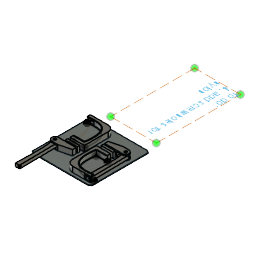
dipoledeployer_v2 (Autodesk Fusion 360 design; units mm, degrees)
Autodesk Fusion 360 part; units mm, degrees
sketch "Sketch1" plane through (0, 0, 0) normal (0, 0, 1) x (1, 0, 0) in component "baseplate"
  line L0 (0, 0) -> (100, 0)
  line L1 (100, 0) -> (100, -100)
  line L2 (100, -100) -> (0, -100)
  line L3 (0, -100) -> (0, 0)
  dimension "d1" = 100
  dimension "d2" = 100
  constraint horizontal L0
  constraint vertical L1
  constraint horizontal L2
  constraint vertical L3
  constraint coincident L0.start L3.end
  measures "d1" distance of L0.start L0.end
  measures "d2" distance of L0.start L2.end
extrude "Extrude1" add sketch "Sketch1" along normal blind 2 makes body 1 in component "baseplate"
sketch "Sketch2" plane through (0, 0, 2) normal (0, 0, 1) x (-1, 0, 0) in component "baseplate"
  line L0 (0, 100) -> (-100, 100)
  line L1 (-100, 100) -> (-100, 0)
  line L2 (-100, 0) -> (0, 0)
  line L3 (0, 0) -> (0, 100)
  line L4 (-50, 0) -> (-50, 100)
  line L5 (0, 50) -> (-100, 50)
  line L6 (-50, 50) -> (-50, 39)
  line L7 (-59, 29) -> (-79, 29)
  line L8 (-79, 29) -> (-79, 35)
  line L9 (-79, 35) -> (-59, 35)
  line L10 (-59, 35) -> (-59, 29)
  line L11 (-59, 37) -> (-79, 37)
  line L12 (-79, 37) -> (-79, 39)
  line L13 (-79, 39) -> (-59, 39)
  line L14 (-59, 39) -> (-59, 37)
  line L15 (-41, 29) -> (-21, 29)
  line L16 (-21, 29) -> (-21, 35)
  line L17 (-21, 35) -> (-41, 35)
  line L18 (-41, 35) -> (-41, 29)
  line L19 (-41, 37) -> (-21, 37)
  line L20 (-41, 39) -> (-41, 37)
  line L21 (-21, 39) -> (-41, 39)
  line L22 (-21, 37) -> (-21, 39)
  line L23 (-41, 71) -> (-21, 71)
  line L24 (-41, 65) -> (-41, 71)
  line L25 (-21, 65) -> (-41, 65)
  line L26 (-21, 71) -> (-21, 65)
  line L27 (-41, 63) -> (-21, 63)
  line L28 (-21, 61) -> (-41, 61)
  line L29 (-21, 63) -> (-21, 61)
  line L30 (-41, 61) -> (-41, 63)
  line L31 (-100, 0) -> (0, 100) construction
  line L32 (0, 0) -> (-100, 100) construction
  dimension "d5" = 20
  dimension "d6" = 6
  dimension "d7" = 9
  dimension "d8" = 15
  dimension "d11" = 2
  dimension "d12" = 20
  dimension "d13" = 2
  dimension "d14" = 9
  constraint midpoint L2 L4.start
  constraint midpoint L0 L4.end
  constraint midpoint L3 L5.start
  constraint midpoint L1 L5.end
  constraint midpoint L5 L6.start
  constraint coincident L4 L6.end
  constraint horizontal L7
  constraint vertical L8
  constraint horizontal L9
  constraint vertical L10
  constraint horizontal L11
  constraint vertical L12
  constraint horizontal L13
  constraint vertical L14
  constraint symmetric L4 L7.start L15.start
  constraint symmetric L4 L7.end L15.end
  constraint symmetric L4 L8.end L16.end
  constraint symmetric L4 L9.end L17.end
  constraint symmetric L4 L11.start L19.start
  constraint symmetric L4 L11.end L19.end
  constraint symmetric L4 L12.end L21.start
  constraint symmetric L4 L13.end L20.start
  constraint symmetric L5 L15.start L23.start
  constraint symmetric L5 L15.end L23.end
  constraint symmetric L5 L16.end L25.start
  constraint symmetric L5 L17.end L24.start
  constraint symmetric L5 L19.start L27.start
  constraint symmetric L5 L19.end L27.end
  constraint symmetric L5 L20.start L28.end
  constraint symmetric L5 L21.start L28.start
  constraint coincident L1.end L2.start
  constraint coincident L0.start L3.end
  constraint coincident L2.end L3.start
  constraint coincident L0.end L1.start
  measures "d5" distance of L7.start L7.end
  measures "d6" distance of L7.start L9.end
  measures "d7" distance of L4 L10
  measures "d8" distance of L5 L9
  measures "d11" distance of L9 L11
  measures "d12" distance of L12.end L13.end
  measures "d13" distance of L11.end L12.end
  measures "d14" distance of L4 L14
extrude "Extrude2" add sketch "Sketch2" along normal blind 15 separate body contours L7 L8 L9 L10 | L11 L12 L13 L14 makes body 2 at (65.6667, -29, 7) makes body 3 at (65.6667, -37, 7) in component "baseplate"
extrude "Extrude3" add sketch "Sketch2" along normal blind 15 contours L7 L8 L9 L10 | L11 L12 L13 L14 | L23 L24 L25 L26 | L27 L28 L29 L30 bodies 1 2 3 in component "baseplate"
sketch "Sketch3" plane through (0, -61, 0) normal (0, 1, 0) x (-1, 0, 0) in component "baseplate"
  line L0 (-41, 2) -> (-21, 2)
  line L1 (-21, 2) -> (-21, 17)
  line L2 (-21, 17) -> (-41, 17)
  line L3 (-41, 17) -> (-41, 2)
  line L4 (-21, 2) -> (-21, 9.5)
  line L5 (-21, 9.5) -> (-41, 9.5)
  line L6 (-31, 9.5) -> (-28, 9.5)
  circle A0 centre (-28, 9.5) radius 1.65
  line L7 (-31, 9.5) -> (-38, 9.5)
  circle A1 centre (-38, 9.5) radius 1.65
  dimension "d17" = 3.3
  dimension "d18" = 3.3
  constraint coincident L0.end L1.start
  constraint midpoint L1 L4.end
  constraint midpoint L3 L5.end
  constraint midpoint L5 L6.start
  constraint coincident L5 L6.end
  constraint coincident L6.end A0.centre
  constraint coincident L5 L7.end
  constraint coincident L7.end A1.centre
  measures "d17" diameter of A0
  measures "d18" diameter of A1
extrude "Extrude4" cut sketch "Sketch3" against normal blind 6 contours L5 L7 A1 | L5 L7 A1 | L5 L6 A0 | L5 L6 A0 bodies 1 in component "baseplate"
sketch "Sketch4" plane through (0, -39, 0) normal (0, -1, 0) x (1, 0, 0) in component "baseplate"
  line L0 (59, 2) -> (79, 2)
  line L1 (79, 2) -> (79, 17)
  line L2 (79, 17) -> (59, 17)
  line L3 (59, 17) -> (59, 2)
  line L4 (59, 17) -> (79, 2)
  line L5 (79, 17) -> (59, 2)
  line L6 (69, 9.5) -> (62, 9.5)
  line L7 (62, 9.5) -> (72, 9.5)
  circle A0 centre (62, 9.5) radius 1.65
  circle A1 centre (72, 9.5) radius 1.65
  dimension "d21" = 3.3
  dimension "d22" = 3.3
  constraint coincident L2.end L3.start
  constraint coincident L0.end L1.start
  constraint coincident L1.end L2.start
  constraint coincident L0.start L3.end
  constraint midpoint L4 L6.start
  constraint horizontal L6
  constraint parallel L6 L7
  constraint coincident L6.end L7.start
  constraint coincident L7.end A1.centre
  measures "d21" diameter of A0
  measures "d22" diameter of A1
extrude "Extrude5" cut sketch "Sketch4" against normal blind 6 contours A0 | A1 bodies 1 in component "baseplate"
sketch "Sketch5" plane through (0, 0, 2) normal (0, 0, 1) x (-1, 0, 0) in component "baseplate"
  line L0 (-21, 71) -> (-21, 65)
  line L1 (-21, 65) -> (-41, 65)
  line L2 (-41, 65) -> (-41, 71)
  line L3 (-41, 71) -> (-21, 71)
  line L4 (-59, 35) -> (-59, 29)
  line L5 (-59, 29) -> (-79, 29)
  line L6 (-79, 29) -> (-79, 35)
  line L7 (-79, 35) -> (-59, 35)
  line L8 (-41, 61) -> (-41, 63)
  line L9 (-41, 63) -> (-21, 63)
  line L10 (-21, 63) -> (-21, 61)
  line L11 (-21, 61) -> (-41, 61)
  line L12 (-59, 39) -> (-59, 37)
  line L13 (-59, 37) -> (-79, 37)
  line L14 (-79, 37) -> (-79, 39)
  line L15 (-79, 39) -> (-59, 39)
  line L16 (0, 100) -> (-100, 100)
  line L17 (-100, 100) -> (-100, 0)
  line L18 (-100, 0) -> (0, 0)
  line L19 (0, 0) -> (0, 100)
sketch "Sketch6" plane through (0, 0, 2) normal (0, 0, 1) x (-1, 0, 0) in component "baseplate"
  line L0 (-79, 35) -> (-89, 35)
  line L1 (-79, 29) -> (-79, 24)
  line L2 (-79, 24) -> (-89, 24)
  arc A0 (-89, 35) -> (-89, 24) centre (-89, 29.5) ccw
  line L3 (-21, 65) -> (-11, 65)
  line L4 (-21, 71) -> (-21, 76)
  line L5 (-21, 76) -> (-11, 76)
  arc A1 (-11, 65) -> (-11, 76) centre (-11, 70.5) ccw
  line L6 (-79, 24) -> (-59, 29)
  line L7 (-21, 76) -> (-41, 71)
  line L8 (-79, 35) -> (-79, 29)
  line L9 (-79, 29) -> (-59, 29)
  line L10 (-21, 71) -> (-21, 65)
  line L11 (-21, 71) -> (-41, 71)
  point P0 (-59, 29)
  point P1 (-41, 71)
  dimension "d33" = 10
  dimension "d34" = 5.5
  constraint horizontal L0
  constraint vertical L1
  constraint perpendicular L1 L2
  constraint tangent L0 A0
  constraint tangent L2 A0
  constraint horizontal L3
  constraint perpendicular L3 L4
  constraint perpendicular L4 L5
  constraint tangent L5 A1
  constraint tangent L3 A1
  constraint perpendicular L0 L8
  constraint perpendicular L1 L9
  constraint perpendicular L3 L10
  constraint perpendicular L4 L11
  constraint coincident P0 L6.end
  constraint coincident P1 L7.end
  measures "d33" distance of L0.start L0.end
  measures "d34" radius of A0
extrude "Extrude6" add sketch "Sketch6" along normal blind 15 bodies 1 in component "baseplate"
extrude "Extrude7" cut sketch "Sketch6" along normal blind 7 from surface at 4 contours L3 L4 L5 A1 L10 bodies 1 in component "baseplate"
extrude "Extrude8" cut sketch "Sketch6" along normal blind 7 from surface at 4 contours L0 L1 L2 A0 L8 bodies 1 in component "baseplate"
sketch "Sketch7" plane through (0, 0, 2) normal (0, 0, 1) x (-1, 0, 0) in component "baseplate"
  line L0 (-11, 65) -> (-41, 65)
  line L1 (-41, 65) -> (-41, 71)
  line L2 (-41, 71) -> (-21, 76)
  line L3 (-21, 76) -> (-11, 76)
  arc A0 (-11, 65) -> (-11, 76) centre (-11, 70.5) ccw
  line L4 (-89, 35) -> (-59, 35)
  line L5 (-59, 35) -> (-59, 29)
  line L6 (-59, 29) -> (-79, 24)
  line L7 (-79, 24) -> (-89, 24)
  arc A1 (-89, 35) -> (-89, 24) centre (-89, 29.5) ccw
  line L8 (-41, 61) -> (-41, 63)
  line L9 (-41, 63) -> (-21, 63)
  line L10 (-21, 63) -> (-21, 61)
  line L11 (-21, 61) -> (-41, 61)
  line L12 (-59, 39) -> (-59, 37)
  line L13 (-59, 37) -> (-79, 37)
  line L14 (-79, 37) -> (-79, 39)
  line L15 (-79, 39) -> (-59, 39)
  line L16 (0, 100) -> (-100, 100)
  line L17 (-100, 100) -> (-100, 0)
  line L18 (-100, 0) -> (0, 0)
  line L19 (0, 0) -> (0, 100)
sketch "Sketch8" plane through (0, 0, 17) normal (0, 0, 1) x (-1, 0, 0) in component "baseplate"
  line L0 (-41, 71) -> (-41, 65)
  line L1 (-41, 65) -> (-11, 65)
  arc A0 (-11, 65) -> (-11, 76) centre (-11, 70.5) ccw
  line L2 (-11, 76) -> (-21, 76)
  line L3 (-21, 76) -> (-41, 71)
  circle A1 centre (-11, 70.5) radius 2.25
  dimension "d35" = 4.5
  constraint concentric A0 A1
  measures "d35" diameter of A1
sketch "Sketch9" plane through (0, 0, 17) normal (0, 0, 1) x (-1, 0, 0) in component "baseplate"
  line L0 (-59, 35) -> (-89, 35)
  arc A0 (-89, 35) -> (-89, 24) centre (-89, 29.5) ccw
  line L1 (-89, 24) -> (-79, 24)
  line L2 (-79, 24) -> (-59, 29)
  line L3 (-59, 29) -> (-59, 35)
  circle A1 centre (-89, 29.5) radius 2.25
  dimension "d36" = 4.5
  constraint concentric A0 A1
  measures "d36" diameter of A1
extrude "Extrude9" cut sketch "Sketch9" sketch "Sketch8" against normal blind 15 contours A1 of sketch 2 contours A1 bodies 1 in component "baseplate"
sketch "Sketch10" plane through (0, 0, 2) normal (0, 0, 1) x (-1, 0, 0) in component "baseplate"
  line L0 (-79, 45) -> (-55, 45)
  line L1 (-55, 45) -> (-55, 85)
  line L2 (-65, 95) -> (-95, 95)
  line L3 (-95, 95) -> (-95, 90)
  line L4 (-79, 45) -> (-79, 50)
  arc A0 (-55, 85) -> (-65, 95) centre (-65, 85) ccw
  line L5 (-79, 50) -> (-60, 50)
  spline S0 degree 5 poles (-60, 50) (-59.7146, 51.8705) (-59.2285, 55.5196) (-58.7531, 60.7176) (-58.6353, 67.0874) (-59.4079, 74.0504) (-61.1872, 79.9198) (-64.0631, 84.5979) (-68.0975, 88.0173) (-73.2633, 90.2075) (-79.4828, 91.2531) (-85.236, 91.2448) (-89.961, 90.7929) (-93.2905, 90.2968) (-95, 90) knots 0 0 0 0 0 0 0.1 0.2 0.3 0.4 0.5 0.6 0.7 0.8 0.9 1 1 1 1 1 1
  line L6 (-50, 0) -> (-50, 100)
  line L7 (-21, 45) -> (-45, 45)
  line L8 (-21, 45) -> (-21, 50)
  line L9 (-21, 50) -> (-40, 50)
  spline S1 degree 5 poles (-40, 50) (-40.2854, 51.8705) (-40.7715, 55.5196) (-41.2469, 60.7176) (-41.3647, 67.0874) (-40.5921, 74.0504) (-38.8128, 79.9198) (-35.9369, 84.5979) (-31.9025, 88.0173) (-26.7367, 90.2075) (-20.5172, 91.2531) (-14.764, 91.2448) (-10.039, 90.7929) (-6.7095, 90.2968) (-5, 90) knots 0 0 0 0 0 0 0.1 0.2 0.3 0.4 0.5 0.6 0.7 0.8 0.9 1 1 1 1 1 1
  line L10 (-61.5241, 40.0105) -> (-58.4759, 59.9895)
  line L11 (-85.1973, 91.7017) -> (-104.8027, 88.2983)
  line L12 (-38.4759, 40.0105) -> (-41.5241, 59.9895)
  line L13 (-14.8027, 91.7017) -> (4.8027, 88.2983)
  line L14 (-45, 45) -> (-45, 85)
  arc A1 (-35, 95) -> (-45, 85) centre (-35, 85) ccw
  line L15 (-35, 95) -> (-5, 95)
  line L16 (-5, 95) -> (-5, 90)
  line L17 (0, 50) -> (-100, 50)
  line L18 (-21, 55) -> (-45, 55)
  line L19 (-45, 55) -> (-45, 15)
  line L20 (-21, 55) -> (-21, 50)
  line L21 (-21, 50) -> (-40, 50)
  spline S2 degree 5 poles (-40, 50) (-40.2854, 48.1295) (-40.7715, 44.4804) (-41.2469, 39.2824) (-41.3647, 32.9126) (-40.5921, 25.9496) (-38.8128, 20.0802) (-35.9369, 15.4021) (-31.9025, 11.9827) (-26.7367, 9.7925) (-20.5172, 8.7469) (-14.764, 8.7552) (-10.039, 9.2071) (-6.7095, 9.7032) (-5, 10) knots 0 0 0 0 0 0 0.1 0.2 0.3 0.4 0.5 0.6 0.7 0.8 0.9 1 1 1 1 1 1
  line L22 (-38.4759, 59.9895) -> (-41.5241, 40.0105)
  line L23 (-14.8027, 8.2983) -> (4.8027, 11.7017)
  arc A2 (-45, 15) -> (-35, 5) centre (-35, 15) ccw
  line L24 (-35, 5) -> (-5, 5)
  line L25 (-5, 5) -> (-5, 10)
  point P0 (-65, 85)
  point P1 (-35, 85)
  point P2 (-35, 15)
  dimension "d39" = 24
  dimension "d40" = 5
  dimension "d41" = 5
  dimension "d42" = 10
  dimension "d43" = 40
  dimension "d44" = 30
  dimension "d45" = 19
  constraint horizontal L0
  constraint perpendicular L0 L1
  constraint perpendicular L1 L2
  constraint perpendicular L2 L3
  constraint perpendicular L0 L4
  constraint tangent L1 A0
  constraint tangent L2 A0
  constraint perpendicular L4 L5
  constraint coincident P0 A0.centre
  constraint midpoint L5.end L10
  constraint midpoint L3.end L11
  constraint symmetric L0.start L6 L7.start
  constraint symmetric L0.end L6 L7.end
  constraint symmetric L2.end L6 L15.end
  constraint symmetric L3.end L6 S1.end
  constraint symmetric L4.end L6 L8.end
  constraint symmetric L1.end L6 L14.end
  constraint symmetric L2.start L6 A1.start
  constraint symmetric A0 L6 A1
  constraint symmetric L5.end L6 L9.end
  constraint symmetric P0 L6 P1
  constraint symmetric L6 L10.start L12.start
  constraint symmetric L6 L10.end L12.end
  constraint symmetric L6 L11.start L13.start
  constraint symmetric L6 L11.end L13.end
  constraint symmetric L7.start L17 L18.start
  constraint symmetric L7.end L17 L18.end
  constraint symmetric L8.end L17 L9.start
  constraint symmetric L9.end L17 S1.start
  constraint symmetric P1 L17 P2
  constraint symmetric S1.end L17 S2.end
  constraint symmetric L12.start L17 L22.start
  constraint symmetric L12.end L17 L22.end
  constraint symmetric L13.start L17 L23.start
  constraint symmetric L13.end L17 L23.end
  constraint symmetric L14.end L17 L19.end
  constraint symmetric A1.start L17 A2.end
  constraint symmetric A1 L17 A2
  constraint symmetric L15.end L17 L24.end
  measures "d39" distance of L0.start L0.end
  measures "d40" distance of L2.end L3.end
  measures "d41" distance of L0.start L4.end
  measures "d42" radius of A0
  measures "d43" distance of L0.end L1.end
  measures "d44" distance of L2.end L2.start
  measures "d45" distance of L4.end L5.end
extrude "Extrude10" add sketch "Sketch10" along normal blind 15 contours L0 L4 L5 L10 L17 | L0 L1 L10 L17 | L1 L2 L3 A0 S0 L17 | L9 L17 L18 L20 L21 L22 | L7 L19 S2 A2 L24 L25 | L7 S2 L22 | S1 L12 L18 | L12 L14 L17 L18 L19 | L7 L14 L17 L19 L22 | S1 L18 L22 bodies 1 in component "baseplate"
sketch "Sketch11" plane through (0, 0, 17) normal (0, 0, 1) x (-1, 0, 0) in component "baseplate"
  line L0 (-79, 45) -> (-55, 45)
  line L1 (-55, 45) -> (-55, 85)
  arc A0 (-55, 85) -> (-65, 95) centre (-65, 85) ccw
  line L2 (-65, 95) -> (-95, 95)
  line L3 (-95, 95) -> (-95, 90)
  spline S0 degree 5 poles (-95, 90) (-93.2905, 90.2968) (-89.961, 90.7929) (-85.236, 91.2448) (-79.4828, 91.2531) (-73.2633, 90.2075) (-68.0975, 88.0173) (-64.0631, 84.5979) (-61.1872, 79.9198) (-59.4079, 74.0504) (-58.6353, 67.0874) (-58.7531, 60.7176) (-59.2285, 55.5196) (-59.7146, 51.8705) (-60, 50) knots -1 -1 -1 -1 -1 -1 -0.9 -0.8 -0.7 -0.6 -0.5 -0.4 -0.3 -0.2 -0.1 0 0 0 0 0 0
  line L4 (-60, 50) -> (-79, 50)
  line L5 (-79, 50) -> (-79, 45)
  line L6 (-95, 95) -> (-85, 95)
  line L7 (-85, 95) -> (-85, 91.0896)
  line L8 (-5, 5) -> (-15, 5)
  line L9 (-15, 5) -> (-15, 9)
  line L10 (-5, 5) -> (-5, 10)
  line L11 (-5, 10) -> (-15, 10)
  line L12 (-15, 10) -> (-15, 9)
  dimension "d48" = 10
  dimension "d49" = 90
  dimension "d50" = 10
  constraint coincident L2.end L3.start
  constraint perpendicular L3 L6
  constraint coincident S0 L7.end
  constraint perpendicular L6 L7
  constraint perpendicular L8 L9
  constraint perpendicular L8 L10
  constraint perpendicular L10 L11
  measures "d48" distance of L2.end L6.end
  measures "d49" angle of L7 L8
  measures "d50" distance of L8.start L8.end
extrude "Extrude11" cut sketch "Sketch11" against normal blind 7 from surface at -4 contours L2 L3 S0 L6 L7 | L8 L9 L10 L11 L12 bodies 1 in component "baseplate"
sketch "Sketch13" plane through (0, 0, 6) normal (0, 0, 1) x (-1, 0, 0) in component "baseplate"
  circle A0 centre (-11, 70.5) radius 2.25
  line L0 (-21, 76) -> (-21, 65)
  line L1 (-21, 65) -> (-11, 65)
  arc A1 (-11, 65) -> (-11, 76) centre (-11, 70.5) ccw
  line L2 (-11, 76) -> (-21, 76)
  circle A2 centre (-11, 70.5) radius 5
  line L3 (-5, 5) -> (-6.0006, 70.5763)
  line L4 (-5, 5) -> (-11.9992, 4.8932)
  spline S0 degree 5 poles (-11.9992, 4.8932) (-11.9252, 6.9328) (-11.7854, 10.9544) (-11.6002, 16.8138) (-11.4027, 24.2745) (-11.2457, 32.964) (-11.1908, 40.9291) (-11.255, 48.049) (-11.4586, 54.1813) (-11.821, 59.1863) (-12.3579, 62.9548) (-12.9282, 64.9707) (-13.4323, 65.9409) (-13.8018, 66.3506) (-13.9949, 66.4962) knots 0 0 0 0 0 0 0.1 0.2 0.3 0.4 0.5 0.6 0.7 0.8 0.9 1 1 1 1 1 1
  point P0 (-11.9992, 60.0714)
  dimension "d54" = 10
  dimension "d55" = 7
  constraint concentric A0 A2
  constraint coincident A2 L3.end
  constraint tangent A2 L3
  constraint perpendicular L3 L4
  constraint coincident A2 S0.end
  measures "d54" diameter of A2
  measures "d55" distance of L3.start L4.end
extrude "Extrude1'" add sketch "Sketch13" along normal blind 6.5 from surface at 0.25 separate body contours L1 A1 A2 L3 S0 | L1 A1 L3 L4 S0 | A2 L3 sketch seen with x (1, 0, 0) y (0, 1, 0) z (0, 0, 1) at (0.3158, -2.7195, 1.082) makes body 4
copy_body "CopyPasteBodies1" bodies 4 makes body 5
move_body "Move1" bodies 5 to x (-1, 0, 0) y (0, -1, 0) z (0, 0, 1) at (100.6316, -105.4389, 0)
copy_body "Body->Comp1" bodies 4 removing the originals makes body 6 in component "arm1"
copy_body "Body->Comp2" bodies 5 removing the originals makes body 7 in component "arm2"
sketch "Sketch1 (2)" plane through (0, 0, 3.082) normal (0, 0, 1) x (-1, 0, 0)
  line L0 (-21.3158, 57.7195) -> (-21.3158, 52.7195)
  line L1 (-21.3158, 52.7195) -> (-40.3158, 52.7195)
  spline S0 degree 5 poles (-40.3158, 52.7195) (-40.6012, 50.8489) (-41.0873, 47.1998) (-41.5627, 42.0019) (-41.6805, 35.632) (-40.9079, 28.669) (-39.1286, 22.7997) (-36.2527, 18.1216) (-32.2183, 14.7022) (-27.0525, 12.5119) (-20.833, 11.4663) (-15.0798, 11.4747) (-10.3547, 11.9266) (-7.0253, 12.4227) (-5.3158, 12.7195) knots 0 0 0 0 0 0 0.1 0.2 0.3 0.4 0.5 0.6 0.7 0.8 0.9 1 1 1 1 1 1
  line L2 (-5.3158, 12.7195) -> (-5.3158, 7.7195)
  line L3 (-5.3158, 7.7195) -> (-35.3158, 7.7195)
  arc A0 (-45.3158, 17.7195) -> (-35.3158, 7.7195) centre (-35.3158, 17.7195) ccw
  line L4 (-45.3158, 17.7195) -> (-45.3158, 57.7195)
  line L5 (-45.3158, 57.7195) -> (-21.3158, 57.7195)
  line L6 (-79.3158, 47.7195) -> (-79.3158, 52.7195)
  line L7 (-79.3158, 52.7195) -> (-60.3158, 52.7195)
  spline S1 degree 5 poles (-60.3158, 52.7195) (-60.0304, 54.59) (-59.5443, 58.2391) (-59.0688, 63.437) (-58.9511, 69.8069) (-59.7237, 76.7699) (-61.503, 82.6392) (-64.3788, 87.3173) (-68.4133, 90.7368) (-73.5791, 92.927) (-79.7986, 93.9726) (-85.5518, 93.9642) (-90.2768, 93.5123) (-93.6062, 93.0162) (-95.3158, 92.7195) knots 0 0 0 0 0 0 0.1 0.2 0.3 0.4 0.5 0.6 0.7 0.8 0.9 1 1 1 1 1 1
  line L8 (-95.3158, 92.7195) -> (-95.3158, 97.7195)
  line L9 (-95.3158, 97.7195) -> (-65.3158, 97.7195)
  arc A1 (-55.3158, 87.7195) -> (-65.3158, 97.7195) centre (-65.3158, 87.7195) ccw
  line L10 (-55.3158, 87.7195) -> (-55.3158, 47.7195)
  line L11 (-55.3158, 47.7195) -> (-79.3158, 47.7195)
  line L12 (-11.3158, 67.7195) -> (-41.3158, 67.7195)
  line L13 (-41.3158, 67.7195) -> (-41.3158, 73.7195)
  line L14 (-41.3158, 73.7195) -> (-21.3158, 78.7195)
  line L15 (-21.3158, 78.7195) -> (-11.3158, 78.7195)
  arc A2 (-11.3158, 67.7195) -> (-11.3158, 78.7195) centre (-11.3158, 73.2195) ccw
  line L16 (-89.3158, 37.7195) -> (-59.3158, 37.7195)
  line L17 (-59.3158, 37.7195) -> (-59.3158, 31.7195)
  line L18 (-59.3158, 31.7195) -> (-79.3158, 26.7195)
  line L19 (-79.3158, 26.7195) -> (-89.3158, 26.7195)
  arc A3 (-89.3158, 37.7195) -> (-89.3158, 26.7195) centre (-89.3158, 32.2195) ccw
  line L20 (-41.3158, 63.7195) -> (-41.3158, 65.7195)
  line L21 (-41.3158, 65.7195) -> (-21.3158, 65.7195)
  line L22 (-21.3158, 65.7195) -> (-21.3158, 63.7195)
  line L23 (-21.3158, 63.7195) -> (-41.3158, 63.7195)
  line L24 (-59.3158, 41.7195) -> (-59.3158, 39.7195)
  line L25 (-59.3158, 39.7195) -> (-79.3158, 39.7195)
  line L26 (-79.3158, 39.7195) -> (-79.3158, 41.7195)
  line L27 (-79.3158, 41.7195) -> (-59.3158, 41.7195)
  line L28 (-0.3158, 102.7195) -> (-100.3158, 102.7195)
  line L29 (-100.3158, 102.7195) -> (-100.3158, 2.7195)
  line L30 (-100.3158, 2.7195) -> (-0.3158, 2.7195)
  line L31 (-0.3158, 2.7195) -> (-0.3158, 102.7195)
sketch "Sketch14" plane through (0, 0, 2) normal (0, 0, 1) x (-1, 0, 0) in component "baseplate"
  line L0 (-50, 50) -> (-47.8211, 74.9049)
  line L1 (-50, 50) -> (-25, 50) construction
  circle A0 centre (-47.8211, 74.9049) radius 2.5
  line L2 (-47.8211, 74.9049) -> (-52.1789, 25.0951)
  circle A1 centre (-52.1789, 25.0951) radius 2.5
  dimension "d68" = 85
  dimension "d69" = 25
  dimension "d70" = 5
  dimension "d71" = 50
  dimension "d72" = 5
  constraint horizontal L1
  constraint coincident L0.end A0.centre
  constraint parallel L0 L2
  constraint coincident L2.end A1.centre
  measures "d68" angle of L0 L1
  measures "d69" distance of L0.start L0.end
  measures "d70" diameter of A0
  measures "d71" distance of L0.end L2.end
  measures "d72" diameter of A1
extrude "Extrude15" cut sketch "Sketch14" against normal blind 2 bodies 1 in component "baseplate"
sketch "Sketch2 (2)" plane through (0, 0, 13.832) normal (0, 0, 1) x (-1, 0, 0)
  circle A0 centre (-89.3158, 32.2195) radius 2.25
  line L0 (-95.3158, 97.7195) -> (-94.3152, 32.1432)
  arc A1 (-94.3152, 32.1432) -> (-86.3209, 36.2233) centre (-89.3158, 32.2195) ccw
  spline S0 degree 5 poles (-86.3209, 36.2233) (-86.514, 36.3689) (-86.8835, 36.7786) (-87.3876, 37.7488) (-87.9579, 39.7647) (-88.4948, 43.5331) (-88.8572, 48.5382) (-89.0608, 54.6705) (-89.125, 61.7904) (-89.0701, 69.7554) (-88.9131, 78.4449) (-88.7156, 85.9057) (-88.5303, 91.7651) (-88.3906, 95.7866) (-88.3166, 97.8263) knots -1 -1 -1 -1 -1 -1 -0.9 -0.8 -0.7 -0.6 -0.5 -0.4 -0.3 -0.2 -0.1 0 0 0 0 0 0
  line L1 (-88.3166, 97.8263) -> (-95.3158, 97.7195)
sketch "Sketch2 (3)" plane through (0, 0, 13.832) normal (0, 0, 1) x (-1, 0, 0) in component "arm2"
  circle A0 centre (-89.3158, 32.2195) radius 2.25
  line L0 (-95.3158, 97.7195) -> (-94.3152, 32.1432)
  arc A1 (-94.3152, 32.1432) -> (-86.3209, 36.2233) centre (-89.3158, 32.2195) ccw
  spline S0 degree 5 poles (-86.3209, 36.2233) (-86.514, 36.3689) (-86.8835, 36.7786) (-87.3876, 37.7488) (-87.9579, 39.7647) (-88.4948, 43.5331) (-88.8572, 48.5382) (-89.0608, 54.6705) (-89.125, 61.7904) (-89.0701, 69.7554) (-88.9131, 78.4449) (-88.7156, 85.9057) (-88.5303, 91.7651) (-88.3906, 95.7866) (-88.3166, 97.8263) knots -1 -1 -1 -1 -1 -1 -0.9 -0.8 -0.7 -0.6 -0.5 -0.4 -0.3 -0.2 -0.1 0 0 0 0 0 0
  line L1 (-88.3166, 97.8263) -> (-95.3158, 97.7195)
  line L2 (-95.3158, 97.7195) -> (-95.27, 94.7198)
  line L3 (-95.3158, 97.7195) -> (-92.3161, 97.7652)
  line L4 (-92.3161, 97.7652) -> (-95.27, 94.7198)
  dimension "d89" = 3
  dimension "d90" = 3
  constraint coincident L0.start L1.end
  constraint perpendicular L1 L2
  constraint coincident L1 L3.end
  measures "d89" distance of L0.start L2.end
  measures "d90" distance of L0.start L3.end
extrude "Extrude1''" cut sketch "Sketch2 (3)" against normal blind 1 from surface at -3 contours L0 L1 L2 L3 L4 bodies 7 in component "arm2"
sketch "Sketch1 (3)" plane through (0, 0, 13.832) normal (0, 0, 1) x (-1, 0, 0) in component "arm1"
  circle A0 centre (-11.3158, 73.2195) radius 2.25
  line L0 (-5.3158, 7.7195) -> (-6.3164, 73.2957)
  arc A1 (-6.3164, 73.2957) -> (-14.3107, 69.2157) centre (-11.3158, 73.2195) ccw
  spline S0 degree 5 poles (-14.3107, 69.2157) (-14.1176, 69.0701) (-13.7481, 68.6604) (-13.244, 67.6902) (-12.6737, 65.6742) (-12.1368, 61.9058) (-11.7743, 56.9007) (-11.5708, 50.7684) (-11.5066, 43.6485) (-11.5615, 35.6835) (-11.7185, 26.994) (-11.916, 19.5332) (-12.1012, 13.6739) (-12.241, 9.6523) (-12.315, 7.6127) knots -1 -1 -1 -1 -1 -1 -0.9 -0.8 -0.7 -0.6 -0.5 -0.4 -0.3 -0.2 -0.1 0 0 0 0 0 0
  line L1 (-12.315, 7.6127) -> (-5.3158, 7.7195)
  line L2 (-5.3158, 7.7195) -> (-5.3616, 10.7191)
  line L3 (-5.3158, 7.7195) -> (-8.3154, 7.6737)
  line L4 (-8.3154, 7.6737) -> (-5.3616, 10.7191)
  dimension "d94" = 3
  dimension "d95" = 3
  constraint coincident L0.start L1.end
  constraint perpendicular L1 L2
  constraint perpendicular L2 L3
  measures "d94" distance of L0.start L2.end
  measures "d95" distance of L0.start L3.end
extrude "Extrude1'''" cut sketch "Sketch1 (3)" against normal blind 1 from surface at -3 contours L0 L1 L2 L3 L4 bodies 6 in component "arm1"
sketch "Sketch15" plane through (-0.3158, 2.7195, 2) normal (0, 0, 1) x (-1, 0, 0) in component "baseplate"
  circle A0 centre (-52.4947, 27.8146) radius 2.5
  circle A1 centre (-48.1369, 77.6243) radius 2.5
  line L0 (-21.3158, 57.7195) -> (-21.3158, 52.7195)
  line L1 (-21.3158, 52.7195) -> (-40.3158, 52.7195)
  spline S0 degree 5 poles (-40.3158, 52.7195) (-40.6012, 50.8489) (-41.0873, 47.1998) (-41.5627, 42.0019) (-41.6805, 35.632) (-40.9079, 28.669) (-39.1286, 22.7997) (-36.2527, 18.1216) (-32.2183, 14.7022) (-27.0525, 12.5119) (-20.833, 11.4663) (-15.0798, 11.4747) (-10.3547, 11.9266) (-7.0253, 12.4227) (-5.3158, 12.7195) knots 0 0 0 0 0 0 0.1 0.2 0.3 0.4 0.5 0.6 0.7 0.8 0.9 1 1 1 1 1 1
  line L2 (-5.3158, 12.7195) -> (-5.3158, 7.7195)
  line L3 (-5.3158, 7.7195) -> (-35.3158, 7.7195)
  arc A2 (-45.3158, 17.7195) -> (-35.3158, 7.7195) centre (-35.3158, 17.7195) ccw
  line L4 (-45.3158, 17.7195) -> (-45.3158, 57.7195)
  line L5 (-45.3158, 57.7195) -> (-21.3158, 57.7195)
  line L6 (-79.3158, 47.7195) -> (-79.3158, 52.7195)
  line L7 (-79.3158, 52.7195) -> (-60.3158, 52.7195)
  spline S1 degree 5 poles (-60.3158, 52.7195) (-60.0304, 54.59) (-59.5443, 58.2391) (-59.0688, 63.437) (-58.9511, 69.8069) (-59.7237, 76.7699) (-61.503, 82.6392) (-64.3788, 87.3173) (-68.4133, 90.7368) (-73.5791, 92.927) (-79.7986, 93.9726) (-85.5518, 93.9642) (-90.2768, 93.5123) (-93.6062, 93.0162) (-95.3158, 92.7195) knots 0 0 0 0 0 0 0.1 0.2 0.3 0.4 0.5 0.6 0.7 0.8 0.9 1 1 1 1 1 1
  line L8 (-95.3158, 92.7195) -> (-95.3158, 97.7195)
  line L9 (-95.3158, 97.7195) -> (-65.3158, 97.7195)
  arc A3 (-55.3158, 87.7195) -> (-65.3158, 97.7195) centre (-65.3158, 87.7195) ccw
  line L10 (-55.3158, 87.7195) -> (-55.3158, 47.7195)
  line L11 (-55.3158, 47.7195) -> (-79.3158, 47.7195)
  line L12 (-11.3158, 67.7195) -> (-41.3158, 67.7195)
  line L13 (-41.3158, 67.7195) -> (-41.3158, 73.7195)
  line L14 (-41.3158, 73.7195) -> (-21.3158, 78.7195)
  line L15 (-21.3158, 78.7195) -> (-11.3158, 78.7195)
  arc A4 (-11.3158, 67.7195) -> (-11.3158, 78.7195) centre (-11.3158, 73.2195) ccw
  line L16 (-89.3158, 37.7195) -> (-59.3158, 37.7195)
  line L17 (-59.3158, 37.7195) -> (-59.3158, 31.7195)
  line L18 (-59.3158, 31.7195) -> (-79.3158, 26.7195)
  line L19 (-79.3158, 26.7195) -> (-89.3158, 26.7195)
  arc A5 (-89.3158, 37.7195) -> (-89.3158, 26.7195) centre (-89.3158, 32.2195) ccw
  line L20 (-41.3158, 63.7195) -> (-41.3158, 65.7195)
  line L21 (-41.3158, 65.7195) -> (-21.3158, 65.7195)
  line L22 (-21.3158, 65.7195) -> (-21.3158, 63.7195)
  line L23 (-21.3158, 63.7195) -> (-41.3158, 63.7195)
  line L24 (-59.3158, 41.7195) -> (-59.3158, 39.7195)
  line L25 (-59.3158, 39.7195) -> (-79.3158, 39.7195)
  line L26 (-79.3158, 39.7195) -> (-79.3158, 41.7195)
  line L27 (-79.3158, 41.7195) -> (-59.3158, 41.7195)
  line L28 (-0.3158, 102.7195) -> (-100.3158, 102.7195)
  line L29 (-100.3158, 102.7195) -> (-100.3158, 2.7195)
  line L30 (-100.3158, 2.7195) -> (-0.3158, 2.7195)
  line L31 (-0.3158, 2.7195) -> (-0.3158, 102.7195)
  line L32 (-0.3158, 2.7195) -> (-2.3158, 2.7195)
  line L33 (-2.3158, 2.7195) -> (-2.3158, 4.7195)
  line L34 (-2.3158, 4.7195) -> (-0.3158, 4.7195)
  line L35 (-0.3158, 4.7195) -> (-0.3158, 2.7195)
  line L36 (-2.3158, 4.7195) -> (-4.3158, 2.7195)
  line L37 (-2.3158, 4.7195) -> (0.5126, 4.7195) construction
  line L38 (-2.3158, 2.7195) -> (-4.3158, 2.7195)
  line L39 (-50.3158, 2.7195) -> (-50.3158, 102.7195)
  line L40 (-98.3158, 4.7195) -> (-96.3158, 2.7195)
  line L41 (-98.3158, 2.7195) -> (-98.3158, 4.7195)
  line L42 (-98.3158, 2.7195) -> (-96.3158, 2.7195)
  line L43 (-100.3158, 2.7195) -> (-98.3158, 2.7195)
  line L44 (-100.3158, 4.7195) -> (-100.3158, 2.7195)
  line L45 (-98.3158, 4.7195) -> (-100.3158, 4.7195)
  line L46 (-0.3158, 52.7195) -> (-100.3158, 52.7195)
  line L47 (-100.3158, 102.7195) -> (-98.3158, 102.7195)
  line L48 (-98.3158, 102.7195) -> (-96.3158, 102.7195)
  line L49 (-98.3158, 100.7195) -> (-96.3158, 102.7195)
  line L50 (-98.3158, 102.7195) -> (-98.3158, 100.7195)
  line L51 (-98.3158, 100.7195) -> (-100.3158, 100.7195)
  line L52 (-100.3158, 100.7195) -> (-100.3158, 102.7195)
  line L53 (-2.3158, 100.7195) -> (-4.3158, 102.7195)
  line L54 (-2.3158, 102.7195) -> (-4.3158, 102.7195)
  line L55 (-2.3158, 102.7195) -> (-2.3158, 100.7195)
  line L56 (-0.3158, 102.7195) -> (-2.3158, 102.7195)
  line L57 (-0.3158, 100.7195) -> (-0.3158, 102.7195)
  line L58 (-2.3158, 100.7195) -> (-0.3158, 100.7195)
  dimension "d99" = 2
  dimension "d100" = 2
  dimension "d101" = 135
  constraint horizontal L32
  constraint vertical L33
  constraint horizontal L34
  constraint vertical L35
  constraint coincident L30.end L31.start
  constraint horizontal L37
  constraint coincident L30 L36.end
  constraint symmetric L30.end L39 L29.end
  constraint symmetric L32.end L39 L41.start
  constraint symmetric L33.end L39 L40.start
  constraint symmetric L34.end L39 L44.start
  constraint symmetric L36.end L39 L40.end
  constraint symmetric L30.end L46 L28.start
  constraint symmetric L32.end L46 L54.start
  constraint symmetric L33.end L46 L53.start
  constraint symmetric L34.end L46 L57.start
  constraint symmetric L36.end L46 L53.end
  constraint symmetric L40.start L46 L49.start
  constraint symmetric L40.end L46 L48.end
  constraint symmetric L41.start L46 L47.end
  constraint symmetric L29.end L46 L28.end
  constraint symmetric L44.start L46 L51.end
  measures "d99" distance of L30.end L32.end
  measures "d100" distance of L30.end L34.end
  measures "d101" angle of L36 L37
extrude "Extrude16" cut sketch "Sketch15" against normal blind 6 contours L30 L40 L41 L42 | L30 L33 L36 L38 | L29 L30 L41 L43 L44 L45 | L30 L31 L32 L33 L34 L35 | L28 L53 L54 L55 | L28 L48 L49 L50 | L28 L31 L55 L56 L57 L58 | L28 L29 L47 L50 L51 L52 bodies 1 in component "baseplate"
extrude "Extrude17" cut 1 faces at (16.5229, -57.9401, 0) along direction (0, 0, 1) blind 0.5 on bodies 1 bodies 1 in component "baseplate"
extrude "Extrude19" add 1 faces at (30.1224, -61, 3.9638) along direction (0, 1, 0) blind 2 on bodies 1 bodies 1 in component "baseplate"
sketch "Sketch4 (2)" plane through (0, 0, 0) normal (0, 0, 1) x (1, 0, 0)
  line L0 (13.0179, 160) -> (13.0179, 18.7039) construction
  line L1 (13.0179, 18.7039) -> (90, 18.7039) construction
  line L2 (90, 18.7039) -> (90, 160) construction
  line L3 (90, 160) -> (13.0179, 160) construction
  dimension "d110" = 10
extrude "Extrude20" cut 4 faces at (18.4167, -70.5, 6) (10.0636, -6.4202, 6) (81.5833, -29.5, 6) (89.9407, -93.5793, 6) along direction (0, 0, -1) blind 2.75 on bodies 1 bodies 1 in component "baseplate"
extrude "Extrude21" add 4 faces at (81.5833, -29.5, 13) (89.9407, -93.5793, 13) (10.0636, -6.4202, 13) (18.4167, -70.5, 13) along direction (0, 0, -1) blind 3.75 on bodies 1 bodies 1 in component "baseplate"
extrude "Extrude22" cut 6 faces at (35.3333, -53.3333, 17) (24.953, -70.0775, 17) (27.6667, -60.3333, 17) (65.6667, -37.6667, 17) (64.6667, -46.6667, 17) (75.047, -29.9225, 17) along direction (0, 0, -1) blind 5.75 on bodies 1 bodies 1 in component "baseplate"
extrude "Extrude2'" cut 1 faces at (9.7227, -19.8097, 13.832) along direction (0, 0, -1) blind 1 on bodies 6 bodies 6 in component "arm1"
extrude "Extrude3'" cut 1 faces at (6.3309, -8.7041, 9.832) along direction (0, 0, -1) blind 0.5 on bodies 6 bodies 6 in component "arm1"
extrude "Extrude23" cut 1 faces at (16.5229, -57.9401, 0.5) along direction (0, 0, 1) blind 0.5 on bodies 1 bodies 1 in component "baseplate"
extrude "Extrude24" cut 1 faces at (16.5229, -57.9401, 1) along direction (0, 0, 1) blind 0.25 on bodies 1 bodies 1 in component "baseplate"
delete_face "DeleteFace2" 1 faces at (72.6786, -38.3333, 7.996) on bodies 1 in component "baseplate"
delete_face "DeleteFace3" 1 faces at (61.1048, -37.6667, 8.114) on bodies 1 in component "baseplate"
delete_face "DeleteFace4" 1 faces at (61.1048, -33.6667, 8.114) on bodies 1 in component "baseplate"
delete_face "DeleteFace5" 1 faces at (71.2473, -33.6667, 8.0317) on bodies 1 in component "baseplate"
delete_face "DeleteFace6" 1 faces at (38.8952, -61.6667, 8.114) on bodies 1 in component "baseplate"
delete_face "DeleteFace7" 1 faces at (26.3521, -60.3333, 9.5822) on bodies 1 in component "baseplate"
delete_face "DeleteFace8" 1 faces at (26.3521, -66.3333, 9.4178) on bodies 1 in component "baseplate"
delete_face "DeleteFace9" 1 faces at (38.8952, -66.3333, 8.114) on bodies 1 in component "baseplate"
extrude "Extrude25" add 1 faces at (72.3333, -39, 5.0833) along direction (0, -1, 0) blind 2 on bodies 1 bodies 1 in component "baseplate"
sketch "Sketch6 (2)" plane through (0, 0, -1.7946) normal (0, 0, 1) x (-1, 0, 0)
  circle A0 centre (-173.3503, 9.3964) radius 2.25
  line L0 (-179.3503, 74.8964) -> (-178.3497, 9.3201)
  arc A1 (-178.3497, 9.3201) -> (-170.3553, 13.4002) centre (-173.3503, 9.3964) ccw
  spline S0 degree 5 poles (-170.3553, 13.4002) (-170.5484, 13.5458) (-170.918, 13.9555) (-171.4221, 14.9257) (-171.9924, 16.9416) (-172.5292, 20.7101) (-172.8917, 25.7151) (-173.0952, 31.8474) (-173.1595, 38.9673) (-173.1046, 46.9324) (-172.9475, 55.6219) (-172.7501, 63.0826) (-172.5648, 68.942) (-172.425, 72.9635) (-172.3511, 75.0032) knots -1 -1 -1 -1 -1 -1 -0.9 -0.8 -0.7 -0.6 -0.5 -0.4 -0.3 -0.2 -0.1 0 0 0 0 0 0
  line L1 (-172.3511, 75.0032) -> (-179.3503, 74.8964)
  line L2 (-178.3695, 10.6201) -> (-175.1888, 4.7466)
  line L3 (-178.3695, 10.6201) -> (-183.3265, 4.9429)
  line L4 (-183.3265, 4.9429) -> (-175.1888, 4.7466)
  constraint coincident L0 L2.start
  constraint coincident A1 L2.end
extrude "Extrude2''" cut sketch "Sketch6 (2)" against normal blind 1 from surface at -2.5 contours L0 A1 L2 sketch seen with x (1, 0, 0) y (0, 1, 0) z (0, 0, 1) at (-84.0345, -22.8231, 15.6265) bodies 7 in component "arm2"
sketch "Sketch7 (2)" plane through (0, 0, 3.082) normal (0, 0, 1) x (-1, 0, 0)
  line L0 (-59.3158, 43.7195) -> (-59.3158, 39.7195)
  line L1 (-59.3158, 39.7195) -> (-79.3158, 39.7195)
  line L2 (-79.3158, 39.7195) -> (-79.3158, 43.7195)
  line L3 (-79.3158, 43.7195) -> (-59.3158, 43.7195)
  line L4 (-41.3158, 61.7195) -> (-41.3158, 65.7195)
  line L5 (-41.3158, 65.7195) -> (-21.3158, 65.7195)
  line L6 (-21.3158, 65.7195) -> (-21.3158, 61.7195)
  line L7 (-21.3158, 61.7195) -> (-41.3158, 61.7195)
  line L8 (-89.3158, 37.7195) -> (-59.3158, 37.7195)
  line L9 (-59.3158, 37.7195) -> (-59.3158, 31.7195)
  line L10 (-59.3158, 31.7195) -> (-79.3158, 26.7195)
  line L11 (-79.3158, 26.7195) -> (-89.3158, 26.7195)
  arc A0 (-89.3158, 37.7195) -> (-89.3158, 26.7195) centre (-89.3158, 32.2195) ccw
  line L12 (-11.3158, 67.7195) -> (-41.3158, 67.7195)
  line L13 (-41.3158, 67.7195) -> (-41.3158, 73.7195)
  line L14 (-41.3158, 73.7195) -> (-21.3158, 78.7195)
  line L15 (-21.3158, 78.7195) -> (-11.3158, 78.7195)
  arc A1 (-11.3158, 67.7195) -> (-11.3158, 78.7195) centre (-11.3158, 73.2195) ccw
  line L16 (-79.3158, 47.7195) -> (-79.3158, 52.7195)
  line L17 (-79.3158, 52.7195) -> (-60.3158, 52.7195)
  spline S0 degree 5 poles (-60.3158, 52.7195) (-60.0304, 54.59) (-59.5443, 58.2391) (-59.0688, 63.437) (-58.9511, 69.8069) (-59.7237, 76.7699) (-61.503, 82.6392) (-64.3788, 87.3173) (-68.4133, 90.7368) (-73.5791, 92.927) (-79.7986, 93.9726) (-85.5518, 93.9642) (-90.2768, 93.5123) (-93.6062, 93.0162) (-95.3158, 92.7195) knots 0 0 0 0 0 0 0.1 0.2 0.3 0.4 0.5 0.6 0.7 0.8 0.9 1 1 1 1 1 1
  line L18 (-95.3158, 92.7195) -> (-95.3158, 97.7195)
  line L19 (-95.3158, 97.7195) -> (-65.3158, 97.7195)
  arc A2 (-55.3158, 87.7195) -> (-65.3158, 97.7195) centre (-65.3158, 87.7195) ccw
  line L20 (-55.3158, 87.7195) -> (-55.3158, 47.7195)
  line L21 (-55.3158, 47.7195) -> (-79.3158, 47.7195)
  line L22 (-21.3158, 57.7195) -> (-21.3158, 52.7195)
  line L23 (-21.3158, 52.7195) -> (-40.3158, 52.7195)
  spline S1 degree 5 poles (-40.3158, 52.7195) (-40.6012, 50.8489) (-41.0873, 47.1998) (-41.5627, 42.0019) (-41.6805, 35.632) (-40.9079, 28.669) (-39.1286, 22.7997) (-36.2527, 18.1216) (-32.2183, 14.7022) (-27.0525, 12.5119) (-20.833, 11.4663) (-15.0798, 11.4747) (-10.3547, 11.9266) (-7.0253, 12.4227) (-5.3158, 12.7195) knots 0 0 0 0 0 0 0.1 0.2 0.3 0.4 0.5 0.6 0.7 0.8 0.9 1 1 1 1 1 1
  line L24 (-5.3158, 12.7195) -> (-5.3158, 7.7195)
  line L25 (-5.3158, 7.7195) -> (-35.3158, 7.7195)
  arc A3 (-45.3158, 17.7195) -> (-35.3158, 7.7195) centre (-35.3158, 17.7195) ccw
  line L26 (-45.3158, 17.7195) -> (-45.3158, 57.7195)
  line L27 (-45.3158, 57.7195) -> (-21.3158, 57.7195)
  circle A4 centre (-48.1369, 77.6243) radius 2.5
  circle A5 centre (-52.4947, 27.8146) radius 2.5
  line L28 (-100.3158, 4.7195) -> (-98.3158, 4.7195)
  line L29 (-98.3158, 4.7195) -> (-96.3158, 2.7195)
  line L30 (-96.3158, 2.7195) -> (-4.3158, 2.7195)
  line L31 (-4.3158, 2.7195) -> (-2.3158, 4.7195)
  line L32 (-2.3158, 4.7195) -> (-0.3158, 4.7195)
  line L33 (-0.3158, 4.7195) -> (-0.3158, 100.7195)
  line L34 (-0.3158, 100.7195) -> (-2.3158, 100.7195)
  line L35 (-2.3158, 100.7195) -> (-4.3158, 102.7195)
  line L36 (-4.3158, 102.7195) -> (-96.3158, 102.7195)
  line L37 (-96.3158, 102.7195) -> (-98.3158, 100.7195)
  line L38 (-98.3158, 100.7195) -> (-100.3158, 100.7195)
  line L39 (-100.3158, 100.7195) -> (-100.3158, 4.7195)
  line L40 (-55.3158, 47.7195) -> (-45.3158, 57.7195)
  line L41 (-55.3158, 57.7195) -> (-45.3158, 47.7195)
  ellipse E0 centre (-50.3158, 52.7195) end of major axis (-50.3158, 65.2195) minor radius 5
  line L42 (-50.3158, 40.2195) -> (-50.3158, 65.2195) construction
  line L43 (-45.3158, 52.7195) -> (-55.3158, 52.7195) construction
  dimension "d131" = 25
  dimension "d132" = 10
  constraint coincident L20.end L21.start
  constraint coincident L26.end L27.start
  constraint coincident L20 L41.start
  constraint coincident L26 L41.end
  constraint perpendicular L40 L41
  constraint coincident E0 L42.start
  constraint coincident E0 L42.end
  constraint coincident E0 L43.start
  constraint coincident E0 L43.end
  constraint midpoint L40 E0.centre
  constraint vertical L42
  measures "d131" distance of E0
extrude "Extrude26" cut sketch "Sketch7 (2)" against normal blind 33 contours L40 L41 E0 | L40 L41 E0 | L40 L41 E0 | L40 L41 E0 sketch seen with x (1, 0, 0) y (0, 1, 0) z (0, 0, 1) at (-0.3158, 2.7195, -1.082) bodies 1 in component "baseplate"
sketch "Sketch9 (2)" plane through (0, 0, 3.082) normal (0, 0, 1) x (-1, 0, 0)
  line L0 (-100.3158, 4.7195) -> (-98.3158, 4.7195)
  line L1 (-98.3158, 4.7195) -> (-96.3158, 2.7195)
  line L2 (-96.3158, 2.7195) -> (-4.3158, 2.7195)
  line L3 (-4.3158, 2.7195) -> (-2.3158, 4.7195)
  line L4 (-2.3158, 4.7195) -> (-0.3158, 4.7195)
  line L5 (-0.3158, 4.7195) -> (-0.3158, 100.7195)
  line L6 (-0.3158, 100.7195) -> (-2.3158, 100.7195)
  line L7 (-2.3158, 100.7195) -> (-4.3158, 102.7195)
  line L8 (-4.3158, 102.7195) -> (-96.3158, 102.7195)
  line L9 (-96.3158, 102.7195) -> (-98.3158, 100.7195)
  line L10 (-98.3158, 100.7195) -> (-100.3158, 100.7195)
  line L11 (-100.3158, 100.7195) -> (-100.3158, 4.7195)
  circle A0 centre (-52.4947, 27.8146) radius 2.5
  circle A1 centre (-48.1369, 77.6243) radius 2.5
  line L12 (-79.3158, 47.7195) -> (-79.3158, 52.7195)
  line L13 (-79.3158, 52.7195) -> (-60.3158, 52.7195)
  spline S0 degree 5 poles (-60.3158, 52.7195) (-60.0304, 54.59) (-59.5443, 58.2391) (-59.0688, 63.437) (-58.9511, 69.8069) (-59.7237, 76.7699) (-61.503, 82.6392) (-64.3788, 87.3173) (-68.4133, 90.7368) (-73.5791, 92.927) (-79.7986, 93.9726) (-85.5518, 93.9642) (-90.2768, 93.5123) (-93.6062, 93.0162) (-95.3158, 92.7195) knots 0 0 0 0 0 0 0.1 0.2 0.3 0.4 0.5 0.6 0.7 0.8 0.9 1 1 1 1 1 1
  line L14 (-95.3158, 92.7195) -> (-95.3158, 97.7195)
  line L15 (-95.3158, 97.7195) -> (-65.3158, 97.7195)
  arc A2 (-55.3158, 87.7195) -> (-65.3158, 97.7195) centre (-65.3158, 87.7195) ccw
  line L16 (-55.3158, 87.7195) -> (-55.3158, 52.7195)
  ellipse E0 centre (-50.3158, 52.7195) end of major axis (-50.3158, 65.2195) minor radius 5 (-45.3158, 52.7195) -> (-55.3158, 52.7195) ccw
  line L17 (-45.3158, 52.7195) -> (-45.3158, 57.7195)
  line L18 (-45.3158, 57.7195) -> (-21.3158, 57.7195)
  line L19 (-21.3158, 57.7195) -> (-21.3158, 52.7195)
  line L20 (-21.3158, 52.7195) -> (-40.3158, 52.7195)
  spline S1 degree 5 poles (-40.3158, 52.7195) (-40.6012, 50.8489) (-41.0873, 47.1998) (-41.5627, 42.0019) (-41.6805, 35.632) (-40.9079, 28.669) (-39.1286, 22.7997) (-36.2527, 18.1216) (-32.2183, 14.7022) (-27.0525, 12.5119) (-20.833, 11.4663) (-15.0798, 11.4747) (-10.3547, 11.9266) (-7.0253, 12.4227) (-5.3158, 12.7195) knots 0 0 0 0 0 0 0.1 0.2 0.3 0.4 0.5 0.6 0.7 0.8 0.9 1 1 1 1 1 1
  line L21 (-5.3158, 12.7195) -> (-5.3158, 7.7195)
  line L22 (-5.3158, 7.7195) -> (-35.3158, 7.7195)
  arc A3 (-45.3158, 17.7195) -> (-35.3158, 7.7195) centre (-35.3158, 17.7195) ccw
  line L23 (-45.3158, 17.7195) -> (-45.3158, 52.7195)
  ellipse E1 centre (-50.3158, 52.7195) end of major axis (-50.3158, 65.2195) minor radius 5 (-55.3158, 52.7195) -> (-45.3158, 52.7195) ccw
  line L24 (-55.3158, 52.7195) -> (-55.3158, 47.7195)
  line L25 (-55.3158, 47.7195) -> (-79.3158, 47.7195)
  line L26 (-11.3158, 67.7195) -> (-41.3158, 67.7195)
  line L27 (-41.3158, 67.7195) -> (-41.3158, 73.7195)
  line L28 (-41.3158, 73.7195) -> (-21.3158, 78.7195)
  line L29 (-21.3158, 78.7195) -> (-11.3158, 78.7195)
  arc A4 (-11.3158, 67.7195) -> (-11.3158, 78.7195) centre (-11.3158, 73.2195) ccw
  line L30 (-89.3158, 37.7195) -> (-59.3158, 37.7195)
  line L31 (-59.3158, 37.7195) -> (-59.3158, 31.7195)
  line L32 (-59.3158, 31.7195) -> (-79.3158, 26.7195)
  line L33 (-79.3158, 26.7195) -> (-89.3158, 26.7195)
  arc A5 (-89.3158, 37.7195) -> (-89.3158, 26.7195) centre (-89.3158, 32.2195) ccw
  line L34 (-41.3158, 61.7195) -> (-41.3158, 65.7195)
  line L35 (-41.3158, 65.7195) -> (-21.3158, 65.7195)
  line L36 (-21.3158, 65.7195) -> (-21.3158, 61.7195)
  line L37 (-21.3158, 61.7195) -> (-41.3158, 61.7195)
  line L38 (-59.3158, 43.7195) -> (-59.3158, 39.7195)
  line L39 (-59.3158, 39.7195) -> (-79.3158, 39.7195)
  line L40 (-79.3158, 39.7195) -> (-79.3158, 43.7195)
  line L41 (-79.3158, 43.7195) -> (-59.3158, 43.7195)
  line L42 (-21.3158, 51.7195) -> (-40.3158, 51.7195)
  spline S2 degree 3 poles (-39.3272, 52.5686) (-40.7364, 43.3321) (-40.921, 35.4407) (-39.693, 29.2259) (-38.6991, 24.196) (-36.7728, 20.3317) (-33.8078, 17.6477) (-30.6734, 14.8106) (-26.3136, 13.2225) (-20.789, 12.7502) (-16.3719, 12.3726) (-11.2442, 12.7053) (-5.4868, 13.7047) knots 0 0 0 0 0.298604 0.298604 0.298604 0.540274 0.540274 0.540274 0.795743 0.795743 0.795743 1 1 1 1
  line L43 (-21.3158, 52.7195) -> (-21.3158, 51.7195)
  line L44 (-5.4868, 13.7047) -> (-5.3158, 12.7195)
  spline S3 degree 3 poles (-61.3044, 52.8703) (-59.8952, 62.1068) (-59.7106, 69.9983) (-60.9386, 76.2131) (-61.9325, 81.2429) (-63.8587, 85.1073) (-66.8238, 87.7912) (-69.9582, 90.6284) (-74.318, 92.2165) (-79.8426, 92.6888) (-84.2597, 93.0664) (-89.3873, 92.7337) (-95.1448, 91.7342) knots 0 0 0 0 0.298604 0.298604 0.298604 0.540274 0.540274 0.540274 0.795743 0.795743 0.795743 1 1 1 1
  line L45 (-79.3158, 53.7195) -> (-60.3158, 53.7195)
  line L46 (-95.3158, 92.7195) -> (-95.1448, 91.7342)
  line L47 (-79.3158, 53.7195) -> (-79.3158, 52.7195)
  dimension "d135" = -1
  dimension "d136" = -1
  dimension "d140" = -1
  dimension "d141" = -1
  constraint coincident L19.end L20.start
  constraint perpendicular L42 L43
  constraint coincident S1.end L21.start
  constraint coincident S0.end L14.start
  constraint coincident L12.end L13.start
  constraint perpendicular L13 L47
extrude "Extrude27" add sketch "Sketch9 (2)" against normal blind 0.5 from surface at 9.25 contours L20 S1 L42 S2 L43 L44 sketch seen with x (1, 0, 0) y (0, 1, 0) z (0, 0, 1) at (-0.3158, 2.7195, -1.082) bodies 1 in component "baseplate"
extrude "Extrude28" add sketch "Sketch9 (2)" against normal blind 0.5 from surface at 9.25 contours L13 S0 S3 L45 L46 L47 sketch seen with x (1, 0, 0) y (0, 1, 0) z (0, 0, 1) at (-0.3158, 2.7195, -1.082) bodies 1 in component "baseplate"
extrude "Extrude30" cut 1 faces at (90.9089, -85.6292, 13.832) faces seen with x (1, 0, 0) y (0, 1, 0) z (0, 0, 1) at (-0.3158, 2.7195, -3.832) along direction (0, 0, -1) blind 1 on bodies 7 bodies 1 in component "baseplate"
extrude "Extrude3''" cut 1 faces at (90.9089, -85.6292, 13.832) along direction (0, 0, -1) blind 1 on bodies 7 bodies 7 in component "arm2"
extrude "Extrude31" cut 1 faces at (80.6674, -29.4515, 9.25) along direction (0, 0, 1) blind 0.5 on bodies 1 bodies 1 in component "baseplate"
extrude "Extrude32" add 1 faces at (88.0956, -33.6314, 10) along direction (0, 0, -1) blind 0.25 on bodies 1 bodies 1 in component "baseplate"
extrude "Extrude33" add 1 faces at (81.5833, -29.5, 9.75) along direction (0, 0, -1) blind 0.5 on bodies 1 bodies 1 in component "baseplate"
component "baseplate" placed x (1, 0, 0) y (0, 1, 0) z (0, 0, 1) at (0.3158, -2.7195, 1.082)
component "arm2" placed x (1, 0, 0) y (0, 1, 0) z (0, 0, 1) at (0, 0, -2.75)
component "arm2" placed x (1, 0, 0) y (0, 1, 0) z (0, 0, 1) at (-78, -41, -2.75)
equation "d111 = 'To do: 4. add screwholes for nylon '"
